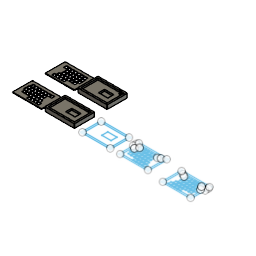
Split_keyboard (Autodesk Fusion 360 design; units mm, degrees)
part number: 2026-04-26-11-28-51-810
Autodesk Fusion 360 part; units mm, degrees
sketch "Sketch1" plane through (0, 0, 0) normal (0, 1, 0) x (1, 0, 0)
  line L0 (-69.957, 50) -> (110.043, 50)
  line L1 (110.043, 50) -> (110.043, -74)
  line L2 (110.043, -74) -> (-69.957, -74)
  line L3 (-69.957, -74) -> (-69.957, 50)
  line L4 (100.043, -64) -> (-59.957, -64)
  line L5 (-59.957, -64) -> (-59.957, 40)
  line L6 (-59.957, 40) -> (100.043, 40)
  line L7 (100.043, 40) -> (100.043, -64)
  line L8 (10, 10) -> (66.0085, 10)
  line L9 (66.0085, 10) -> (66.0085, -26)
  line L10 (66.0085, -26) -> (10, -26)
  line L11 (10, -26) -> (10, 10)
  line L12 (-67, -68) -> (-63, -68)
  line L13 (-63, -68) -> (-63, -72)
  line L14 (-63, -72) -> (-67, -72)
  line L15 (-67, -72) -> (-67, -68)
  line L16 (107, -72) -> (103, -72)
  line L17 (103, -72) -> (103, -68)
  line L18 (103, -68) -> (107, -68)
  line L19 (107, -68) -> (107, -72)
  line L20 (107, 43) -> (103, 43)
  line L21 (103, 43) -> (103, 47)
  line L22 (103, 47) -> (107, 47)
  line L23 (107, 47) -> (107, 43)
  line L24 (-63, 47) -> (-67, 47)
  line L25 (-67, 47) -> (-67, 43)
  line L26 (-67, 43) -> (-63, 43)
  line L27 (-63, 43) -> (-63, 47)
  point P0 (-65, -70)
  point P1 (105, -70)
  point P2 (105, 45)
  point P3 (-65, 45)
  dimension "d2" = 124
  dimension "d3" = 10
  dimension "d6" = 36
  dimension "d79" = 180
  dimension "d80" = 104
  constraint horizontal L0
  constraint vertical L1
  constraint horizontal L2
  constraint vertical L3
  constraint horizontal L8
  constraint vertical L9
  constraint horizontal L10
  constraint vertical L11
  constraint horizontal L12
  constraint vertical L13
  constraint horizontal L14
  constraint vertical L15
  constraint horizontal L16
  constraint vertical L17
  constraint horizontal L18
  constraint vertical L19
  constraint horizontal L20
  constraint vertical L21
  constraint horizontal L22
  constraint vertical L23
  constraint horizontal L24
  constraint vertical L25
  constraint horizontal L26
  constraint vertical L27
  measures "d2" distance of L0.start L2.end
  measures "d6" distance of L8.start L10.end
  measures "d79" distance of L1.end L2.end
  measures "d80" distance of L4.end L5.end
extrude "Extrude3" add sketch "Sketch1" along normal blind 5 contours L0 L1 L2 L3 | L4 L5 L6 L7 | L8 L9 L10 L11 | L12 L13 L14 L15 | L16 L17 L18 L19 | L20 L21 L22 L23 | L24 L25 L26 L27 makes body 1
extrude "Extrude5" add sketch "Sketch1" along normal blind 15 separate body contours L0 L1 L2 L3 | L4 L5 L6 L7 | L12 L13 L14 L15 | L16 L17 L18 L19 | L20 L21 L22 L23 | L24 L25 L26 L27 makes body 2
extrude "Extrude6" add sketch "Sketch1" along normal blind 25 separate body contours L0 L1 L2 L3 | L12 L13 L14 L15 | L16 L17 L18 L19 | L20 L21 L22 L23 | L24 L25 L26 L27 makes body 3
combine "Combine1" operation add target body 3 tool bodies 2 1
hole "Hole1" at (-65, 0, 70) at (-65, 0, -45) at (105, 0, -45) at (105, 0, 70) direction (0, 1, 0) diameter 2 end through all bodies 3
extrude "Extrude7" add sketch "Sketch1" along normal blind 3 separate body contours L12 L13 L14 L15 | L16 L17 L18 L19 | L20 L21 L22 L23 | L24 L25 L26 L27 makes body 4 at (-65.6667, 0, 69.3333) makes body 5 at (105.6667, 0, 70.6667) makes body 6 at (-65.6667, 0, -45.6667) makes body 7 at (105.6667, 0, -44.3333)
combine "Combine2" operation cut target body 3 tool bodies 6 5 4 7
fillet "Fillet1" radius 2 4 edges at (110.043, 12.5, 74) (110.043, 12.5, -50) (-69.957, 12.5, -50) (-69.957, 12.5, 74) on bodies 3
copy_body "CopyPasteBodies1" bodies 3 makes body 8
move_body "Move3" bodies 8 to x (1, 0, 0) y (0, 1, 0) z (0, 0, 1) at (230, 0, 0)
move_body "Move4" bodies 8 to x (1, 0, 0) y (0, 1, 0) z (0, 0, 1) at (0, 0, -200)
sketch "Sketch3" plane through (0, 0, 0) normal (0, 1, 0) x (1, 0, 0)
  line L0 (159.9992, 50) -> (339.9992, 50)
  line L1 (339.9992, 50) -> (339.9992, -74)
  line L2 (339.9992, -74) -> (159.9992, -74)
  line L3 (159.9992, -74) -> (159.9992, 50)
  line L4 (159.9992, 50) -> (159.9992, 33)
  line L5 (183.5, 31) -> (199.5, 31)
  line L6 (199.5, 31) -> (199.5, 15.0011)
  line L7 (199.5, 15.0011) -> (183.5, 15.0011)
  line L8 (183.5, 15.0011) -> (183.5, 31)
  line L9 (202.55, 31) -> (218.5387, 31)
  line L10 (218.5387, 31) -> (218.5387, 15)
  line L11 (218.5387, 15) -> (202.55, 15)
  line L12 (202.55, 15) -> (202.55, 31)
  line L13 (221.6, 31) -> (237.6, 31)
  line L14 (237.6, 31) -> (237.6, 15)
  line L15 (237.6, 15) -> (221.6, 15)
  line L16 (221.6, 15) -> (221.6, 31)
  line L17 (199.5, 15.0011) -> (183.5, 15.0011)
  line L18 (237.6, 15) -> (221.6, 15)
  line L19 (199.5, 31) -> (199.5, 15.0011)
  line L20 (221.6, 15) -> (221.6, 31)
  line L21 (183.5, 31) -> (199.5, 31)
  line L22 (218.5387, 15) -> (202.55, 15)
  line L23 (221.6, 31) -> (237.6, 31)
  line L24 (218.5387, 31) -> (218.5387, 15)
  line L25 (202.55, 31) -> (218.5387, 31)
  line L26 (202.55, 15) -> (202.55, 31)
  line L27 (237.6, 31) -> (237.6, 15)
  line L28 (183.5, 15.0011) -> (183.5, 31)
  line L29 (240.65, 31.0009) -> (256.65, 31.0009)
  line L30 (256.65, 31.0009) -> (256.65, 14.974)
  line L31 (256.65, 14.974) -> (240.65, 14.974)
  line L32 (240.65, 14.974) -> (240.65, 31.0009)
  line L33 (259.7, 31) -> (275.7198, 31)
  line L34 (275.7198, 31) -> (275.7198, 15)
  line L35 (275.7198, 15) -> (259.7, 15)
  line L36 (259.7, 15) -> (259.7, 31)
  line L37 (278.75, 31) -> (294.75, 31)
  line L38 (294.75, 31) -> (294.75, 15)
  line L39 (294.75, 15) -> (278.75, 15)
  line L40 (278.75, 15) -> (278.75, 31)
  line L41 (298.25, 23) -> (298.25, 32)
  line L42 (298.25, 32) -> (312.85, 32)
  line L43 (298.25, 32) -> (313, 32)
  line L44 (313, 32) -> (313, 14)
  line L45 (313, 14) -> (298.25, 14)
  line L46 (298.25, 14) -> (298.25, 32)
  line L47 (159.9992, 50) -> (159.9992, 14)
  line L48 (178.5, 4) -> (178.5, 12)
  line L49 (178.5, 12) -> (194.4987, 12)
  line L50 (194.4987, 12) -> (194.4987, -4)
  line L51 (194.4987, -4) -> (178.5, -4)
  line L52 (178.5, -4) -> (178.5, 12)
  line L53 (197.5, 12) -> (213.5, 12)
  line L54 (213.5, 12) -> (213.5, -4.0185)
  line L55 (213.5, -4.0185) -> (197.5, -4.0185)
  line L56 (197.5, -4.0185) -> (197.5, 12)
  line L57 (216.6, 12.055) -> (232.6304, 12.055)
  line L58 (232.6304, 12.055) -> (232.6304, -3.945)
  line L59 (232.6304, -3.945) -> (216.6, -3.945)
  line L60 (216.6, -3.945) -> (216.6, 12.055)
  line L61 (235.65, 12) -> (251.65, 12)
  line L62 (251.65, 12) -> (251.65, -4.0008)
  line L63 (251.65, -4.0008) -> (235.65, -4.0008)
  line L64 (235.65, -4.0008) -> (235.65, 12)
  line L65 (254.7, 12.0057) -> (270.7123, 12.0057)
  line L66 (270.7123, 12.0057) -> (270.7123, -3.9943)
  line L67 (270.7123, -3.9943) -> (254.7, -3.9943)
  line L68 (254.7, -3.9943) -> (254.7, 12.0057)
  line L69 (273.75, 12.0057) -> (289.8279, 12.0057)
  line L70 (289.8279, 12.0057) -> (289.8279, -3.9943)
  line L71 (289.8279, -3.9943) -> (273.75, -3.9943)
  line L72 (273.75, -3.9943) -> (273.75, 12.0057)
  line L73 (251.65, -7.05) -> (251.65, -23.0508)
  line L74 (235.65, -7.05) -> (251.65, -7.05)
  line L75 (235.65, -23.0508) -> (235.65, -7.05)
  line L76 (251.65, -23.0508) -> (235.65, -23.0508)
  line L77 (270.7123, -23.0443) -> (254.7, -23.0443)
  line L78 (254.7, -23.0443) -> (254.7, -7.0443)
  line L79 (254.7, -7.0443) -> (270.7123, -7.0443)
  line L80 (273.75, -23.0443) -> (273.75, -7.0443)
  line L81 (273.75, -7.0443) -> (289.8279, -7.0443)
  line L82 (270.7123, -7.0443) -> (270.7123, -23.0443)
  line L83 (289.8279, -23.0443) -> (273.75, -23.0443)
  line L84 (289.8279, -7.0443) -> (289.8279, -23.0443)
  line L85 (232.6304, -6.995) -> (232.6304, -22.995)
  line L86 (216.6, -6.995) -> (232.6304, -6.995)
  line L87 (232.6304, -22.995) -> (216.6, -22.995)
  line L88 (216.6, -22.995) -> (216.6, -6.995)
  line L89 (213.5, -7.05) -> (213.5, -23.0685)
  line L90 (197.5, -7.05) -> (213.5, -7.05)
  line L91 (197.5, -23.0685) -> (197.5, -7.05)
  line L92 (213.5, -23.0685) -> (197.5, -23.0685)
  line L93 (194.4987, -7.05) -> (194.4987, -23.05)
  line L94 (178.5, -7.05) -> (194.4987, -7.05)
  line L95 (194.4987, -23.05) -> (178.5, -23.05)
  line L96 (178.5, -23.05) -> (178.5, -7.05)
  line L97 (260.65, -26.1) -> (260.65, -42.1008)
  line L98 (244.65, -26.1) -> (260.65, -26.1)
  line L99 (244.65, -42.1008) -> (244.65, -26.1)
  line L100 (260.65, -42.1008) -> (244.65, -42.1008)
  line L101 (279.7123, -42.0943) -> (263.7, -42.0943)
  line L102 (263.7, -42.0943) -> (263.7, -26.0943)
  line L103 (263.7, -26.0943) -> (279.7123, -26.0943)
  line L104 (282.75, -42.0943) -> (282.75, -26.0943)
  line L105 (282.75, -26.0943) -> (298.8279, -26.0943)
  line L106 (279.7123, -26.0943) -> (279.7123, -42.0943)
  line L107 (298.8279, -42.0943) -> (282.75, -42.0943)
  line L108 (298.8279, -26.0943) -> (298.8279, -42.0943)
  line L109 (241.6304, -26.045) -> (241.6304, -42.045)
  line L110 (225.6, -26.045) -> (241.6304, -26.045)
  line L111 (241.6304, -42.045) -> (225.6, -42.045)
  line L112 (225.6, -42.045) -> (225.6, -26.045)
  line L113 (222.5, -26.1) -> (222.5, -42.1185)
  line L114 (206.5, -26.1) -> (222.5, -26.1)
  line L115 (206.5, -42.1185) -> (206.5, -26.1)
  line L116 (222.5, -42.1185) -> (206.5, -42.1185)
  line L117 (203.4987, -26.1) -> (203.4987, -42.1)
  line L118 (187.5, -26.1) -> (203.4987, -26.1)
  line L119 (203.4987, -42.1) -> (187.5, -42.1)
  line L120 (187.5, -42.1) -> (187.5, -26.1)
  line L121 (252.1304, -45.095) -> (252.1304, -61.095)
  line L122 (252.1304, -61.095) -> (236.1, -61.095)
  line L123 (236.1, -61.095) -> (236.1, -45.095)
  line L124 (255.15, -45.15) -> (271.15, -45.15)
  line L125 (255.15, -61.1508) -> (255.15, -45.15)
  line L126 (271.15, -61.1508) -> (255.15, -61.1508)
  line L127 (271.15, -45.15) -> (271.15, -61.1508)
  line L128 (274.2, -61.1443) -> (274.2, -45.1443)
  line L129 (274.2, -45.1443) -> (290.2123, -45.1443)
  line L130 (290.2123, -61.1443) -> (274.2, -61.1443)
  line L131 (290.2123, -45.1443) -> (290.2123, -61.1443)
  line L132 (293.25, -61.1443) -> (293.25, -45.1443)
  line L133 (293.25, -45.1443) -> (309.3279, -45.1443)
  line L134 (309.3279, -45.1443) -> (309.3279, -61.1443)
  line L135 (309.3279, -61.1443) -> (293.25, -61.1443)
  line L136 (236.1, -45.095) -> (252.1304, -45.095)
  line L137 (169.9992, 40) -> (329.9992, 40)
  line L138 (329.9992, 40) -> (329.9992, -64)
  line L139 (329.9992, -64) -> (169.9992, -64)
  line L140 (169.9992, -64) -> (169.9992, 40)
  line L141 (183.5, 31) -> (183.5, 15.0011)
  line L142 (191.5, 23.0006) -> (169.9992, 23.0006)
  line L143 (555.4, -1.2239, -0.1827) -> (555.4, 14.7761, -0.1827)
  line L144 (539.4, 14.7761, -0.1827) -> (539.4, -1.2239, -0.1827)
  line L145 (447.0008, 23.7761, -0.1827) -> (447.0008, -80.2239, -0.1827)
  line L146 (498.25, -1.2239, -0.1827) -> (498.25, 14.7761, -0.1827)
  line L147 (501.2802, 14.7761, -0.1827) -> (501.2802, -1.2239, -0.1827)
  line L148 (520.35, 14.777, -0.1827) -> (520.35, -1.2499, -0.1827)
  line L149 (478.75, 6.7761, -0.1827) -> (478.75, 15.7761, -0.1827)
  line L150 (539.4, 14.7761, -0.1827) -> (539.4, -1.2239, -0.1827)
  line L151 (437.0008, 33.7761, -0.1827) -> (437.0008, -90.2239, -0.1827)
  line L152 (464, 15.7761, -0.1827) -> (464, -2.2239, -0.1827)
  line L153 (555.4, -1.2239, -0.1827) -> (555.4, 14.7761, -0.1827)
  line L154 (487.1721, -20.2182, -0.1827) -> (503.25, -20.2182, -0.1827)
  line L155 (497.2877, -42.3182, -0.1827) -> (497.2877, -58.3182, -0.1827)
  line L156 (494.25, -42.3182, -0.1827) -> (478.1721, -42.3182, -0.1827)
  line L157 (506.2877, -23.2682, -0.1827) -> (506.2877, -39.2682, -0.1827)
  line L158 (502.8, -77.3682, -0.1827) -> (502.8, -61.3682, -0.1827)
  line L159 (483.75, -61.3682, -0.1827) -> (467.6721, -61.3682, -0.1827)
  line L160 (486.7877, -61.3682, -0.1827) -> (486.7877, -77.3682, -0.1827)
  line L161 (582.5013, -39.2739, -0.1827) -> (598.5, -39.2739, -0.1827)
  line L162 (574.45, -1.2239, -0.1827) -> (574.45, 14.7761, -0.1827)
  line L163 (585.5, 6.7767, -0.1827) -> (607.0008, 6.7767, -0.1827)
  line L164 (589.5, -58.3239, -0.1827) -> (589.5, -42.3239, -0.1827)
  line L165 (570.5, -42.3239, -0.1827) -> (554.5, -42.3239, -0.1827)
  line L166 (582.5013, -4.2239, -0.1827) -> (582.5013, -20.2239, -0.1827)
  line L167 (579.5, -39.2924, -0.1827) -> (579.5, -23.2739, -0.1827)
  line L168 (574.45, 14.7761, -0.1827) -> (558.4613, 14.7761, -0.1827)
  line L169 (617.0008, -90.2239, -0.1827) -> (617.0008, 33.7761, -0.1827)
  line L170 (607.0008, 23.7761, -0.1827) -> (447.0008, 23.7761, -0.1827)
  line L171 (570.5, -58.3424, -0.1827) -> (570.5, -42.3239, -0.1827)
  line L172 (563.5, -23.2739, -0.1827) -> (563.5, -39.2924, -0.1827)
  line L173 (554.5, -58.3424, -0.1827) -> (570.5, -58.3424, -0.1827)
  line L174 (579.5, -20.2424, -0.1827) -> (579.5, -4.2239, -0.1827)
  line L175 (598.5, -23.2739, -0.1827) -> (582.5013, -23.2739, -0.1827)
  line L176 (577.5, -1.2228, -0.1827) -> (593.5, -1.2228, -0.1827)
  line L177 (577.5, 14.7761, -0.1827) -> (577.5, -1.2228, -0.1827)
  line L178 (517.3, -1.2239, -0.1827) -> (517.3, 14.7761, -0.1827)
  line L179 (563.5, -39.2924, -0.1827) -> (579.5, -39.2924, -0.1827)
  line L180 (558.4613, 14.7761, -0.1827) -> (558.4613, -1.2239, -0.1827)
  line L181 (558.4613, -1.2239, -0.1827) -> (574.45, -1.2239, -0.1827)
  line L182 (437.0008, -90.2239, -0.1827) -> (617.0008, -90.2239, -0.1827)
  line L183 (447.0008, -80.2239, -0.1827) -> (607.0008, -80.2239, -0.1827)
  line L184 (563.5, -4.2239, -0.1827) -> (563.5, -20.2424, -0.1827)
  line L185 (598.5, -4.2239, -0.1827) -> (582.5013, -4.2239, -0.1827)
  line L186 (574.45, 14.7761, -0.1827) -> (558.4613, 14.7761, -0.1827)
  line L187 (558.4613, -1.2239, -0.1827) -> (574.45, -1.2239, -0.1827)
  line L188 (617.0008, 33.7761, -0.1827) -> (437.0008, 33.7761, -0.1827)
  line L189 (582.5013, -20.2239, -0.1827) -> (598.5, -20.2239, -0.1827)
  line L190 (540.9, -77.3189, -0.1827) -> (540.9, -61.3189, -0.1827)
  line L191 (554.5, -42.3239, -0.1827) -> (554.5, -58.3424, -0.1827)
  line L192 (544.3696, -39.2189, -0.1827) -> (560.4, -39.2189, -0.1827)
  line L193 (544.3696, -23.2189, -0.1827) -> (544.3696, -39.2189, -0.1827)
  line L194 (525.35, -23.2739, -0.1827) -> (525.35, -39.2747, -0.1827)
  line L195 (525.35, -20.2247, -0.1827) -> (541.35, -20.2247, -0.1827)
  line L196 (544.3696, -20.1689, -0.1827) -> (560.4, -20.1689, -0.1827)
  line L197 (560.4, -23.2189, -0.1827) -> (544.3696, -23.2189, -0.1827)
  line L198 (551.4, -58.2689, -0.1827) -> (551.4, -42.2689, -0.1827)
  line L199 (532.35, -58.3247, -0.1827) -> (532.35, -42.3239, -0.1827)
  line L200 (560.4, -4.1689, -0.1827) -> (544.3696, -4.1689, -0.1827)
  line L201 (563.5, -20.2424, -0.1827) -> (579.5, -20.2424, -0.1827)
  line L202 (577.5, 14.7761, -0.1827) -> (577.5, -1.2228, -0.1827)
  line L203 (593.5, -1.2228, -0.1827) -> (593.5, 14.7761, -0.1827)
  line L204 (593.5, 14.7761, -0.1827) -> (577.5, 14.7761, -0.1827)
  line L205 (593.5, 14.7761, -0.1827) -> (593.5, -1.2228, -0.1827)
  line L206 (593.5, 14.7761, -0.1827) -> (577.5, 14.7761, -0.1827)
  line L207 (617.0008, 33.7761, -0.1827) -> (617.0008, 16.7761, -0.1827)
  line L208 (617.0008, 33.7761, -0.1827) -> (617.0008, -2.2239, -0.1827)
  line L209 (607.0008, -80.2239, -0.1827) -> (607.0008, 23.7761, -0.1827)
  line L210 (582.5013, -23.2739, -0.1827) -> (582.5013, -39.2739, -0.1827)
  line L211 (577.5, -1.2228, -0.1827) -> (593.5, -1.2228, -0.1827)
  line L212 (593.5, -1.2228, -0.1827) -> (593.5, 14.7761, -0.1827)
  line L213 (598.5, -12.2239, -0.1827) -> (598.5, -4.2239, -0.1827)
  line L214 (573.5013, -58.3239, -0.1827) -> (589.5, -58.3239, -0.1827)
  line L215 (589.5, -42.3239, -0.1827) -> (573.5013, -42.3239, -0.1827)
  line L216 (574.45, -1.2239, -0.1827) -> (574.45, 14.7761, -0.1827)
  line L217 (573.5013, -42.3239, -0.1827) -> (573.5013, -58.3239, -0.1827)
  line L218 (579.5, -4.2239, -0.1827) -> (563.5, -4.2239, -0.1827)
  line L219 (598.5, -20.2239, -0.1827) -> (598.5, -4.2239, -0.1827)
  line L220 (579.5, -23.2739, -0.1827) -> (563.5, -23.2739, -0.1827)
  line L221 (598.5, -39.2739, -0.1827) -> (598.5, -23.2739, -0.1827)
  line L222 (558.4613, 14.7761, -0.1827) -> (558.4613, -1.2239, -0.1827)
  line L223 (478.75, -2.2239, -0.1827) -> (478.75, 15.7761, -0.1827)
  line L224 (536.35, -1.2499, -0.1827) -> (536.35, 14.777, -0.1827)
  line L225 (513.3, -58.3182, -0.1827) -> (513.3, -42.3182, -0.1827)
  line L226 (522.3, -20.2182, -0.1827) -> (522.3, -4.2182, -0.1827)
  line L227 (560.4, -20.1689, -0.1827) -> (560.4, -4.1689, -0.1827)
  line L228 (539.4, -1.2239, -0.1827) -> (555.4, -1.2239, -0.1827)
  line L229 (541.35, -23.2739, -0.1827) -> (525.35, -23.2739, -0.1827)
  line L230 (521.85, -77.3747, -0.1827) -> (521.85, -61.3739, -0.1827)
  line L231 (541.35, -4.2239, -0.1827) -> (525.35, -4.2239, -0.1827)
  line L232 (544.3696, -4.1689, -0.1827) -> (544.3696, -20.1689, -0.1827)
  line L233 (525.35, -4.2239, -0.1827) -> (525.35, -20.2247, -0.1827)
  line L234 (516.35, -58.3247, -0.1827) -> (532.35, -58.3247, -0.1827)
  line L235 (525.35, -39.2747, -0.1827) -> (541.35, -39.2747, -0.1827)
  line L236 (532.35, -42.3239, -0.1827) -> (516.35, -42.3239, -0.1827)
  line L237 (520.35, -1.2499, -0.1827) -> (536.35, -1.2499, -0.1827)
  line L238 (535.3696, -42.2689, -0.1827) -> (535.3696, -58.2689, -0.1827)
  line L239 (516.35, -42.3239, -0.1827) -> (516.35, -58.3247, -0.1827)
  line L240 (505.85, -61.3739, -0.1827) -> (505.85, -77.3747, -0.1827)
  line L241 (502.8, -61.3682, -0.1827) -> (486.7877, -61.3682, -0.1827)
  line L242 (478.1721, -42.3182, -0.1827) -> (478.1721, -58.3182, -0.1827)
  line L243 (482.25, -1.2239, -0.1827) -> (498.25, -1.2239, -0.1827)
  line L244 (503.25, -20.2182, -0.1827) -> (503.25, -4.2182, -0.1827)
  line L245 (503.25, -4.2182, -0.1827) -> (487.1721, -4.2182, -0.1827)
  line L246 (506.2877, -4.2182, -0.1827) -> (506.2877, -20.2182, -0.1827)
  line L247 (464, -2.2239, -0.1827) -> (478.75, -2.2239, -0.1827)
  line L248 (467.6721, -77.3682, -0.1827) -> (483.75, -77.3682, -0.1827)
  line L249 (503.25, -23.2682, -0.1827) -> (487.1721, -23.2682, -0.1827)
  line L250 (478.1721, -58.3182, -0.1827) -> (494.25, -58.3182, -0.1827)
  line L251 (487.1721, -23.2682, -0.1827) -> (487.1721, -39.2682, -0.1827)
  line L252 (535.3696, -58.2689, -0.1827) -> (551.4, -58.2689, -0.1827)
  line L253 (487.1721, -39.2682, -0.1827) -> (503.25, -39.2682, -0.1827)
  line L254 (467.6721, -61.3682, -0.1827) -> (467.6721, -77.3682, -0.1827)
  line L255 (483.75, -77.3682, -0.1827) -> (483.75, -61.3682, -0.1827)
  line L256 (503.25, -39.2682, -0.1827) -> (503.25, -23.2682, -0.1827)
  line L257 (486.7877, -77.3682, -0.1827) -> (502.8, -77.3682, -0.1827)
  line L258 (494.25, -58.3182, -0.1827) -> (494.25, -42.3182, -0.1827)
  line L259 (487.1721, -4.2182, -0.1827) -> (487.1721, -20.2182, -0.1827)
  line L260 (522.3, -39.2682, -0.1827) -> (522.3, -23.2682, -0.1827)
  line L261 (541.35, -39.2747, -0.1827) -> (541.35, -23.2739, -0.1827)
  line L262 (540.9, -61.3189, -0.1827) -> (524.8696, -61.3189, -0.1827)
  line L263 (539.4, -1.2239, -0.1827) -> (555.4, -1.2239, -0.1827)
  line L264 (524.8696, -61.3189, -0.1827) -> (524.8696, -77.3189, -0.1827)
  line L265 (560.4, -39.2189, -0.1827) -> (560.4, -23.2189, -0.1827)
  line L266 (541.35, -20.2247, -0.1827) -> (541.35, -4.2239, -0.1827)
  line L267 (551.4, -42.2689, -0.1827) -> (535.3696, -42.2689, -0.1827)
  line L268 (524.8696, -77.3189, -0.1827) -> (540.9, -77.3189, -0.1827)
  line L269 (522.3, -23.2682, -0.1827) -> (506.2877, -23.2682, -0.1827)
  line L270 (505.85, -77.3747, -0.1827) -> (521.85, -77.3747, -0.1827)
  line L271 (555.4, 14.7761, -0.1827) -> (539.4, 14.7761, -0.1827)
  line L272 (536.35, 14.777, -0.1827) -> (520.35, 14.777, -0.1827)
  line L273 (482.25, 14.7761, -0.1827) -> (482.25, -1.2239, -0.1827)
  line L274 (478.75, 15.7761, -0.1827) -> (464, 15.7761, -0.1827)
  line L275 (478.75, 15.7761, -0.1827) -> (464.15, 15.7761, -0.1827)
  line L276 (498.25, 14.7761, -0.1827) -> (482.25, 14.7761, -0.1827)
  line L277 (513.3, -42.3182, -0.1827) -> (497.2877, -42.3182, -0.1827)
  line L278 (501.2802, -1.2239, -0.1827) -> (517.3, -1.2239, -0.1827)
  line L279 (555.4, 14.7761, -0.1827) -> (539.4, 14.7761, -0.1827)
  line L280 (506.2877, -39.2682, -0.1827) -> (522.3, -39.2682, -0.1827)
  line L281 (497.2877, -58.3182, -0.1827) -> (513.3, -58.3182, -0.1827)
  line L282 (517.3, 14.7761, -0.1827) -> (501.2802, 14.7761, -0.1827)
  line L283 (522.3, -4.2182, -0.1827) -> (506.2877, -4.2182, -0.1827)
  line L284 (506.2877, -20.2182, -0.1827) -> (522.3, -20.2182, -0.1827)
  line L285 (521.85, -61.3739, -0.1827) -> (505.85, -61.3739, -0.1827)
  point P0 (165, -70)
  point P1 (335, -70)
  point P2 (335, 45)
  point P3 (165, 45)
  point P4 (442, -86.2239)
  point P5 (442, 28.7761)
  point P6 (612, -86.2239)
  point P7 (612, 28.7761)
  dimension "d23" = 124
  dimension "d24" = 17
  dimension "d56" = 36
  dimension "d82" = 180
  dimension "d83" = 10
  dimension "d84" = 21.5008
  dimension "d96" = 124
  dimension "d97" = 17
  dimension "d98" = 36
  dimension "d99" = 180
  dimension "d100" = 21.5008
  constraint horizontal L0
  constraint vertical L1
  constraint horizontal L2
  constraint vertical L3
  constraint perpendicular L0 L4
  constraint horizontal L5
  constraint vertical L6
  constraint horizontal L7
  constraint vertical L8
  constraint horizontal L9
  constraint vertical L10
  constraint horizontal L11
  constraint vertical L12
  constraint horizontal L13
  constraint vertical L14
  constraint horizontal L15
  constraint vertical L16
  constraint horizontal L21
  constraint vertical L19
  constraint horizontal L17
  constraint vertical L28
  constraint horizontal L25
  constraint vertical L24
  constraint horizontal L22
  constraint vertical L26
  constraint horizontal L23
  constraint vertical L27
  constraint horizontal L18
  constraint vertical L20
  constraint horizontal L29
  constraint vertical L30
  constraint horizontal L31
  constraint vertical L32
  constraint horizontal L33
  constraint vertical L34
  constraint horizontal L35
  constraint vertical L36
  constraint horizontal L37
  constraint vertical L38
  constraint horizontal L39
  constraint vertical L40
  constraint perpendicular L41 L42
  constraint horizontal L43
  constraint vertical L44
  constraint horizontal L45
  constraint vertical L46
  constraint perpendicular L0 L47
  constraint horizontal L49
  constraint vertical L50
  constraint horizontal L51
  constraint vertical L52
  constraint horizontal L53
  constraint vertical L54
  constraint horizontal L55
  constraint vertical L56
  constraint horizontal L57
  constraint vertical L58
  constraint horizontal L59
  constraint vertical L60
  constraint horizontal L61
  constraint vertical L62
  constraint horizontal L63
  constraint vertical L64
  constraint horizontal L65
  constraint vertical L66
  constraint horizontal L67
  constraint vertical L68
  constraint horizontal L69
  constraint vertical L70
  constraint horizontal L71
  constraint vertical L72
  constraint horizontal L94
  constraint vertical L93
  constraint horizontal L95
  constraint vertical L96
  constraint horizontal L90
  constraint vertical L89
  constraint horizontal L92
  constraint vertical L91
  constraint horizontal L86
  constraint vertical L85
  constraint horizontal L87
  constraint vertical L88
  constraint horizontal L74
  constraint vertical L73
  constraint horizontal L76
  constraint vertical L75
  constraint horizontal L79
  constraint vertical L82
  constraint horizontal L77
  constraint vertical L78
  constraint horizontal L81
  constraint vertical L84
  constraint horizontal L83
  constraint vertical L80
  constraint horizontal L118
  constraint vertical L117
  constraint horizontal L119
  constraint vertical L120
  constraint horizontal L114
  constraint vertical L113
  constraint horizontal L116
  constraint vertical L115
  constraint horizontal L110
  constraint vertical L109
  constraint horizontal L111
  constraint vertical L112
  constraint horizontal L98
  constraint vertical L97
  constraint horizontal L100
  constraint vertical L99
  constraint horizontal L103
  constraint vertical L106
  constraint horizontal L101
  constraint vertical L102
  constraint horizontal L105
  constraint vertical L108
  constraint horizontal L107
  constraint vertical L104
  constraint horizontal L136
  constraint vertical L121
  constraint horizontal L122
  constraint vertical L123
  constraint horizontal L124
  constraint vertical L127
  constraint horizontal L126
  constraint vertical L125
  constraint horizontal L129
  constraint vertical L131
  constraint horizontal L130
  constraint vertical L128
  constraint horizontal L133
  constraint vertical L134
  constraint horizontal L135
  constraint vertical L132
  constraint coincident L140 L142.end
  constraint perpendicular L140 L142
  measures "d23" distance of L0.start L2.end
  measures "d24" distance of L0.start L4.end
  measures "d56" distance of L0.start L47.end
  measures "d82" distance of L1.end L2.end
  measures "d84" distance of L142.start L142.end
move_body "Move5" bodies 3 to x (1, 0, 0) y (0, 1, 0) z (0, 0, 1) at (-220, 0, 0)
extrude "Extrude9" add sketch "Sketch3" along normal blind 3 separate body contours L0 L1 L2 L3 L4 L47 | L137 L138 L139 L140 makes body 9
hole "Hole2" at (165, 0, -45) at (335, 0, -45) at (335, 0, 70) at (165, 0, 70) direction (0, 1, 0) diameter 2 end through all bodies 9
move_body "Move6" bodies 9 to x (1, 0, 0) y (0, 1, 0) z (0, 0, 1) at (-450, 25, 0)
fillet "Fillet2" radius 2 4 edges at (-110.0008, 26.5, 74) (-110.0008, 26.5, -50) (-290.0008, 26.5, -50) (-290.0008, 26.5, 74) on bodies 9
fillet "Fillet3" radius 1 8 edges at (-110.5866, 28, 73.4142) (-110.0008, 28, 12) (-110.5866, 28, -49.4142) (-200.0008, 28, -50) (-289.415, 28, -49.4142) (-290.0008, 28, 12) (-289.415, 28, 73.4142) (-200.0008, 28, 74) on bodies 9
extrude "Extrude12" add sketch "Sketch3" along normal blind 3 separate body contours L145 L170 L183 L209 | L151 L169 L182 L188 L207 L208 in plane through (0, -0.1827, 0) normal (0, 1, 0) makes body 10
hole "Hole6" at (442, -0.1827, -28.7761) at (442, -0.1827, 86.2239) at (612, -0.1827, 86.2239) at (612, -0.1827, -28.7761) direction (0, 1, 0) diameter 2 end through all bodies 10
move_body "Move12" bodies 10 to x (1, 0, 0) y (0, 1, 0) z (0, 0, 1) at (-275, 25, -216)
move_body "Move13" bodies 10 to x (1, 0, 0) y (0, 1, 0) z (0, 0, 1) at (-2, 0, 0)
fillet "Fillet6" radius 2 4 edges at (160.0008, 26.3173, -125.7761) (340.0008, 26.3173, -125.7761) (340.0008, 26.3173, -249.7761) (160.0008, 26.3173, -249.7761) on bodies 10
fillet "Fillet7" radius 1 8 edges at (339.415, 27.8173, -126.3619) (340.0008, 27.8173, -187.7761) (339.415, 27.8173, -249.1903) (250.0008, 27.8173, -249.7761) (160.5866, 27.8173, -249.1903) (160.0008, 27.8173, -187.7761) (160.5866, 27.8173, -126.3619) (250.0008, 27.8173, -125.7761) on bodies 10
move_body "Move14" bodies 10 8 to x (1, 0, 0) y (0, 1, 0) z (0, 0, 1) at (-450, 0, 0)
move_body "Move15" bodies 8 10 to x (1, 0, 0) y (0, 1, 0) z (0, 0, 1) at (250, 0, 0)
sketch "Sketch4" plane through (0, 0, 0) normal (0, 1, 0) x (1, 0, 0)
  line L0 (270, 90) -> (261.5, 90)
  line L1 (261.5, 90) -> (261.5, 110)
  line L2 (261.5, 110) -> (270, 110)
  line L3 (270, 110) -> (270, 90)
  dimension "d125" = 20
  constraint horizontal L0
  constraint vertical L1
  constraint horizontal L2
  constraint vertical L3
  measures "d125" distance of L0.start L2.end
extrude "Extrude13" add sketch "Sketch4" along normal blind 3 separate body makes body 11
copy_body "CopyPasteBodies2" bodies 11 makes body 12
move_body "Move16" bodies 12 to x (1, 0, 0) y (0, 1, 0) z (0, 0, 1) at (17, 0, 0)
move_body "Move17" bodies 11 to x (1, 0, 0) y (0, 1, 0) z (0, 0, 1) at (-154, 13, -149)
combine "Combine3" operation cut target body 8 tool bodies 11
move_body "Move18" bodies 12 to x (1, 0, 0) y (0, 1, 0) z (0, 0, 1) at (-431, 12, 53)
combine "Combine4" operation cut target body 3 tool bodies 12
move_body "Move19" bodies 8 to x (1, 0, 0) y (0, 1, 0) z (0, 0, 1) at (-250, 0, 0)
move_body "Move20" bodies 9 to x (1, 0, 0) y (0, 1, 0) z (0, 0, 1) at (-200, -25, 0)
move_body "Move21" bodies 10 to x (1, 0, 0) y (0, 1, 0) z (0, 0, 1) at (-450, -25, 0)
extrude "Extrude14" add sketch "Sketch4" along normal blind 3 separate body makes body 13
move_body "Move22" bodies 13 to x (1, 0, 0) y (0, 1, 0) z (0, 0, 1) at (-14, 0, 0)
copy_body "CopyPasteBodies3" bodies 13 makes body 14
move_body "Move23" bodies 14 to x (1, 0, 0) y (0, 1, 0) z (0, 0, 1) at (-12, 0, 0)
copy_body "CopyPasteBodies4" bodies 14 makes body 15
move_body "Move24" bodies 15 to x (1, 0, 0) y (0, 1, 0) z (0, 0, 1) at (-12, 0, 0)
copy_body "CopyPasteBodies5" bodies 15 makes body 16
move_body "Move25" bodies 16 to x (1, 0, 0) y (0, 1, 0) z (0, 0, 1) at (-11, 0, 0)
move_body "Move26" bodies 16 to x (1, 0, 0) y (0, 1, 0) z (0, 0, 1) at (-355, 13, -140)
combine "Combine5" operation add target body 8 tool bodies 16
move_body "Move27" bodies 15 to x (1, 0, 0) y (0, 1, 0) z (0, 0, 1) at (-375, 19, -144)
combine "Combine6" operation cut target body 8 tool bodies 15
move_body "Move28" bodies 13 to x (1, 0, 0) y (0, 1, 0) z (0, 0, 1) at (-400, 12, 60)
combine "Combine7" operation add target body 13 tool bodies 3
move_body "Move29" bodies 14 to x (1, 0, 0) y (0, 1, 0) z (0, 0, 1) at (-380, 15, 57)
move_body "Move30" bodies 14 to x (1, 0, 0) y (0, 1, 0) z (0, 0, 1) at (0, 2, 0)
combine "Combine8" operation cut target body 13 tool bodies 14
